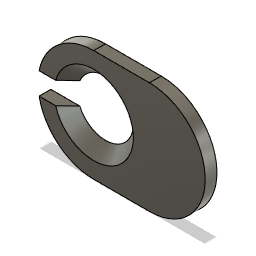
socket (Autodesk Fusion 360 design; units mm, degrees)
Autodesk Fusion 360 part; units mm, degrees
sketch "Sketch1" plane through (0, 0, 0) normal (0, 0, 1) x (1, 0, 0)
  arc A0 (2, 0.1) -> (2, 3.9) centre (2, 2) ccw
  line L0 (2, 0.1) -> (0.1, 0.1)
  line L1 (2, 3.9) -> (0.1, 3.9)
  line L2 (-0.7729, 1.625) -> (-1.7626, 1.625)
  line L3 (-1.7626, 2.375) -> (-0.7729, 2.375)
  arc A1 (0.1, 3.9) -> (-1.7626, 2.375) centre (0.1, 2) ccw
  arc A2 (-1.7626, 1.625) -> (0.1, 0.1) centre (0.1, 2) ccw
  arc A3 (-0.7729, 1.625) -> (-0.7729, 2.375) centre (0.1, 2) ccw
  line L4 (0, 0) -> (10, 0) construction
  dimension "d1" = 3.8
  dimension "d2" = 3.8
  dimension "d3" = 1.9
  dimension "jointrad" = 1.9
  dimension "d5" = 0.375
  dimension "d6" = 0.75
  dimension "ypos" = 2
  dimension "xpos" = 2
  dimension "d17" = 10
  dimension "jointangle" = 180
  constraint coincident L0.end A1
  constraint tangent L0 A1
  constraint tangent A0 L1
  constraint tangent A0 L0
  constraint tangent L1 A1
  constraint coincident L0 A2.end
  constraint concentric A1 A3
  constraint coincident L2.end A1
  constraint concentric A1 A2
  constraint parallel L1 L3
  constraint coincident L4.start origin
  constraint horizontal L4
  measures "d1" diameter of A0
  measures "d2" diameter of A1
  measures "d3" distance of A0.centre A1.centre
  measures "jointrad" diameter of A3
  measures "d5" distance of A0.centre L2
  measures "d6" distance of L2 L3
  measures "ypos" vertical distance of A0.centre L4.start
  measures "xpos" horizontal distance of A0.centre L4.start
  measures "d17" distance of L4.start L4.end
  measures "jointangle" angle of L3 L4
extrude "Extrude1" add sketch "Sketch1" along normal blind 0.4
chamfer "Chamfer1" distance 0.4 angle 45 1 edges at (1.05, 2, 0.4)
equation "d1 = jointrad * 2"
equation "d2 = d1"
equation "d3 = jointrad"
equation "d5 = ( 0.75 / 2 ) * 1 mm"
equation "d6 = d5 * 2"
equation "jointdepth = 0.4 mm"
equation "d11 = jointdepth"
